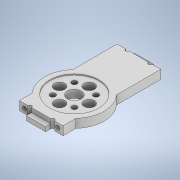
# Autodesk Inventor part: Leg_joint_yaw_frame
Saved by Autodesk Inventor 2020 (Build 240168000, 168)
## iProperties
Created: 2021-10-29
Part Number: Leg_joint_yaw_frame
Material: 一般
Document SubType Name: Modeling
Designer: Masato Kubotera
Density: 1 g/cm^3
Appearance: 既定
Author: Masato Kubotera
Autodesk Inventor part; units mm, degrees
ref_plane "YZ Plane" through (0, 0, 0) normal (1, 0, 0) x (0, 1, 0)
ref_plane "XZ Plane" through (0, 0, 0) normal (0, 1, 0) x (-1, 0, 0)
ref_plane "XY Plane" through (0, 0, 0) normal (0, 0, 1) x (1, 0, 0)
derived "Inner_support_stand.ipt"
sketch "スケッチ1" plane through (0, 0, 0) normal (0, 0, 1) x (1, 0, 0)
  circle A0 centre (0, 0) radius 13.95 construction
  line L0 (0, 13.95) -> (0, -13.95) construction
  circle A1 centre (0, 8.5) radius 1.35 construction
  circle A2 centre (-8.5, 0) radius 1.35 construction
  circle A3 centre (0, -8.5) radius 1.35 construction
  circle A4 centre (8.5, 0) radius 1.35 construction
  circle A5 centre (0, 0) radius 5 construction
  circle A6 centre (0, 0) radius 5.01 construction
  circle A7 centre (-6.1872, 6.1872) radius 2.25 construction
  line L1 (-9.8641, 9.8641) -> (9.8641, -9.8641) construction
  circle A8 centre (-6.1872, 6.1872) radius 1.55
  line L2 (-9.2656, 5.3623) -> (-8.9938, 6.3766) construction
  line L3 (-8.4407, 8.4407) -> (-7.4265, 8.7125) construction
  line L4 (-5.3623, 9.2656) -> (-4.6199, 8.5231) construction
  line L5 (-3.1088, 7.012) -> (-3.3806, 5.9978) construction
  line L6 (-3.9337, 3.9337) -> (-4.9479, 3.6619) construction
  line L7 (-7.012, 3.1088) -> (-7.7545, 3.8513) construction
  circle A9 centre (0, 0) radius 12.49 construction
  arc A10 (-7.4265, 8.7125) -> (-8.7125, 7.4265) centre (-7.6983, 7.6983) ccw construction
  arc A11 (-8.9938, 6.3766) -> (-8.5231, 4.6199) centre (-8.2513, 5.6341) ccw construction
  arc A12 (-7.7545, 3.8513) -> (-5.9978, 3.3806) centre (-6.7403, 4.123) ccw construction
  arc A13 (-4.9479, 3.6619) -> (-3.6619, 4.9479) centre (-4.6761, 4.6761) ccw construction
  arc A14 (-3.3806, 5.9978) -> (-3.8513, 7.7545) centre (-4.123, 6.7403) ccw construction
  arc A15 (-4.6199, 8.5231) -> (-6.3766, 8.9938) centre (-5.6341, 8.2513) ccw construction
  line L8 (-6.3766, 8.9938) -> (-5.3623, 9.2656) construction
  line L9 (-7.4265, 8.7125) -> (-6.3766, 8.9938) construction
  line L10 (-4.6199, 8.5231) -> (-3.8513, 7.7545) construction
  line L11 (-3.8513, 7.7545) -> (-3.1088, 7.012) construction
  line L12 (-3.3806, 5.9978) -> (-3.6619, 4.9479) construction
  line L13 (-3.6619, 4.9479) -> (-3.9337, 3.9337) construction
  line L14 (-4.9479, 3.6619) -> (-5.9978, 3.3806) construction
  line L15 (-5.9978, 3.3806) -> (-7.012, 3.1088) construction
  line L16 (-7.7545, 3.8513) -> (-8.5231, 4.6199) construction
  line L17 (-8.5231, 4.6199) -> (-9.2656, 5.3623) construction
  line L18 (-8.9938, 6.3766) -> (-8.7125, 7.4265) construction
  line L19 (-8.7125, 7.4265) -> (-8.4407, 8.4407) construction
  circle A16 centre (-8.5, 0) radius 2.55 construction
  line L20 (-8.7125, -7.4265) -> (-8.9938, -6.3766) construction
  circle A17 centre (-6.1872, -6.1872) radius 2.25 construction
  circle A18 centre (-6.1872, -6.1872) radius 1.55
  circle A19 centre (0, -8.5) radius 2.55 construction
  arc A20 (-3.8513, -7.7545) -> (-3.3806, -5.9978) centre (-4.123, -6.7403) ccw construction
  line L21 (-3.6619, -4.9479) -> (-3.3806, -5.9978) construction
  arc A21 (-3.6619, -4.9479) -> (-4.9479, -3.6619) centre (-4.6761, -4.6761) ccw construction
  line L22 (-5.9978, -3.3806) -> (-4.9479, -3.6619) construction
  arc A22 (-5.9978, -3.3806) -> (-7.7545, -3.8513) centre (-6.7403, -4.123) ccw construction
  line L23 (-8.5231, -4.6199) -> (-7.7545, -3.8513) construction
  arc A23 (-8.5231, -4.6199) -> (-8.9938, -6.3766) centre (-8.2513, -5.6341) ccw construction
  arc A24 (-8.7125, -7.4265) -> (-7.4265, -8.7125) centre (-7.6983, -7.6983) ccw construction
  line L24 (-6.3766, -8.9938) -> (-7.4265, -8.7125) construction
  arc A25 (-6.3766, -8.9938) -> (-4.6199, -8.5231) centre (-5.6341, -8.2513) ccw construction
  line L25 (-3.8513, -7.7545) -> (-4.6199, -8.5231) construction
  line L26 (7.4265, -8.7125) -> (6.3766, -8.9938) construction
  circle A26 centre (6.1872, -6.1872) radius 2.25 construction
  circle A27 centre (6.1872, -6.1872) radius 1.55
  circle A28 centre (8.5, 0) radius 2.55 construction
  arc A29 (7.7545, -3.8513) -> (5.9978, -3.3806) centre (6.7403, -4.123) ccw construction
  line L27 (4.9479, -3.6619) -> (5.9978, -3.3806) construction
  arc A30 (4.9479, -3.6619) -> (3.6619, -4.9479) centre (4.6761, -4.6761) ccw construction
  line L28 (3.3806, -5.9978) -> (3.6619, -4.9479) construction
  arc A31 (3.3806, -5.9978) -> (3.8513, -7.7545) centre (4.123, -6.7403) ccw construction
  line L29 (4.6199, -8.5231) -> (3.8513, -7.7545) construction
  arc A32 (4.6199, -8.5231) -> (6.3766, -8.9938) centre (5.6341, -8.2513) ccw construction
  arc A33 (7.4265, -8.7125) -> (8.7125, -7.4265) centre (7.6983, -7.6983) ccw construction
  line L30 (8.9938, -6.3766) -> (8.7125, -7.4265) construction
  arc A34 (8.9938, -6.3766) -> (8.5231, -4.6199) centre (8.2513, -5.6341) ccw construction
  line L31 (7.7545, -3.8513) -> (8.5231, -4.6199) construction
  line L32 (8.7125, 7.4265) -> (8.9938, 6.3766) construction
  circle A35 centre (6.1872, 6.1872) radius 2.25 construction
  circle A36 centre (6.1872, 6.1872) radius 1.55
  circle A37 centre (0, 8.5) radius 2.55 construction
  arc A38 (3.8513, 7.7545) -> (3.3806, 5.9978) centre (4.123, 6.7403) ccw construction
  line L33 (3.6619, 4.9479) -> (3.3806, 5.9978) construction
  arc A39 (3.6619, 4.9479) -> (4.9479, 3.6619) centre (4.6761, 4.6761) ccw construction
  line L34 (5.9978, 3.3806) -> (4.9479, 3.6619) construction
  arc A40 (5.9978, 3.3806) -> (7.7545, 3.8513) centre (6.7403, 4.123) ccw construction
  line L35 (8.5231, 4.6199) -> (7.7545, 3.8513) construction
  arc A41 (8.5231, 4.6199) -> (8.9938, 6.3766) centre (8.2513, 5.6341) ccw construction
  arc A42 (8.7125, 7.4265) -> (7.4265, 8.7125) centre (7.6983, 7.6983) ccw construction
  line L36 (6.3766, 8.9938) -> (7.4265, 8.7125) construction
  arc A43 (6.3766, 8.9938) -> (4.6199, 8.5231) centre (5.6341, 8.2513) ccw construction
  line L37 (3.8513, 7.7545) -> (4.6199, 8.5231) construction
  line L38 (-8.8318, 8.8318) -> (-3.5426, 3.5426) construction
  circle A44 centre (0, 0) radius 4
  line L39 (-12.5, -19) -> (-12.5, -11.5954)
  line L40 (-12.5, 37) -> (-7.6, 37)
  line L41 (-12.5, -19) -> (12.5, 37) construction
  line L42 (-12.5, 37) -> (12.5, -19) construction
  arc A45 (-12.5, 11.5954) -> (-12.5, -11.5954) centre (0, 0) ccw
  circle A46 centre (0, 0) radius 14.05
  line L43 (-12.5, 11.5954) -> (-12.5, 37)
  circle A47 centre (0, 8.5) radius 3
  circle A48 centre (-8.5, 0) radius 3
  circle A49 centre (0, -8.5) radius 3
  circle A50 centre (8.5, 0) radius 3
  line L44 (-5.5, -19) -> (-5.5, -22)
  line L45 (-5.5, -22) -> (5.5, -22)
  arc A51 (-5.5, -19) -> (-7.6, -19) centre (-6.55, -19) ccw
  line L46 (-7.6, -19) -> (-12.5, -19)
  line L47 (-5.5, 37) -> (-5.5, 39.9)
  line L48 (-5.5, 39.9) -> (5.5, 39.9)
  arc A52 (-7.6, 37) -> (-5.5, 37) centre (-6.55, 37) ccw
  line L49 (-5.5, -19) -> (5.5, -19)
  line L50 (-5.5, 37) -> (5.5, 37)
  line L51 (0, -22) -> (0, 39.9) construction
  line L52 (12.5, -19) -> (12.5, -11.5954)
  line L53 (12.5, 11.5954) -> (12.5, 37)
  arc A53 (7.6, -19) -> (5.5, -19) centre (6.55, -19) ccw
  arc A54 (5.5, 37) -> (7.6, 37) centre (6.55, 37) ccw
  line L54 (12.5, 37) -> (7.6, 37)
  arc A55 (12.5, -11.5954) -> (12.5, 11.5954) centre (0, 0) ccw
  line L55 (5.5, -19) -> (5.5, -22)
  line L56 (7.6, -19) -> (12.5, -19)
  line L57 (5.5, 37) -> (5.5, 39.9)
  point P0 (-7.012, 3.1088)
  point P1 (-3.9337, 3.9337)
  point P2 (-3.1088, 7.012)
  point P3 (-3.1088, -7.012)
  point P4 (-3.9337, -3.9337)
  point P5 (-7.012, -3.1088)
  point P6 (-9.2656, -5.3623)
  point P7 (-8.4407, -8.4407)
  point P8 (-5.3623, -9.2656)
  point P9 (7.012, -3.1088)
  point P10 (3.9337, -3.9337)
  point P11 (3.1088, -7.012)
  point P12 (5.3623, -9.2656)
  point P13 (8.4407, -8.4407)
  point P14 (9.2656, -5.3623)
  point P15 (3.1088, 7.012)
  point P16 (3.9337, 3.9337)
  point P17 (7.012, 3.1088)
  point P18 (9.2656, 5.3623)
  point P19 (8.4407, 8.4407)
  point P20 (5.3623, 9.2656)
  point P21 (-9.2318, 8.3532)
  point P22 (-9.2318, -8.3532)
  point P23 (-8.3532, -9.2318)
  point P24 (8.3532, -9.2318)
  point P25 (9.2318, -8.3532)
  point P26 (9.2318, 8.3532)
  point P27 (8.3532, 9.2318)
  point P28 (-8.3532, 9.2318)
  point P29 (0, 9)
  dimension "d2" = 25
  dimension "d5" = 3
  dimension "d6" = 0.1
  dimension "d7" = 6
  dimension "d10" = 360
  dimension "d12" = 1.05
  dimension "d13" = 11
  dimension "d14" = 3
  dimension "d15" = 1.05
  dimension "d16" = 2.9
  dimension "d17" = 11
  dimension "d40" = 19
  dimension "d41" = 56
  dimension "d42" = 25
  measures "d2" distance of L40.start L41.end
  measures "d5" radial gap between concentric circles of A45 A46
  measures "d6" radial gap between concentric circles of A46 A0
  measures "d7" diameter of A47
  measures "d12" radius of A51
  measures "d13" distance of L45.end L44.end
  measures "d14" distance of L44.end L44.start
  measures "d15" radius of A52
  measures "d16" distance of L47.start L47.end
  measures "d17" distance of L47.end L48.end
  measures "d40" distance from line of L49 point (0, 0)
  measures "d41" distance between parallel lines of L46 L40
  measures "d42" distance between parallel lines of L52 L39
extrude "押し出し1" add sketch "スケッチ1" along normal blind 5 contours L39 A45 L43 L40 A52 L50 A54 L54 L53 A55 L52 L56 A53 L49 A51 L46
extrude "押し出し2" add sketch "スケッチ1" along normal blind 2.5 contours L49 L55 L45 L44 | L47 L48 L57 L50
extrude "押し出し3" add sketch "スケッチ1" along normal blind 4.5 contours A46
sketch "スケッチ2" plane through (-7.6, -19, 5) normal (0, -1, 0) x (-1, 0, 0)
  line L0 (4.9, 5) -> (0, 5) projected
  line L1 (6.45, 0) -> (-21.65, 0) projected
  line L2 (-7.6, 0) -> (-7.6, 5) construction
  point P0 (1.9, 2.5)
  point P1 (-17.1, 2.5)
  dimension "d24" = 2.5
  dimension "d25" = 19
  constraints: 2 end point, 1 midpoint, 1 symmetric about line, 1 vertical
  measures "d24" distance from line of L0 point (1.9, 2.5)
  measures "d25" distance of point (-17.1, 2.5) point (1.9, 2.5)
hole "穴1" at (-9.5, -19, 2.5) at (9.5, -19, 2.5) direction (0, 1, 0) diameter 2.459 depth 4 tip angle 118 thread size "M3x0.5" class "6H" standard "ISO Metric profile"
sketch "スケッチ3" plane through (7.6, 37, 0) normal (0, 1, 0) x (1, 0, 0)
  circle A0 centre (1.9, -2.5) radius 1.2295 projected
  circle A1 centre (-17.1, -2.5) radius 1.2295 projected
  point P0 (-7.6, 0)
  constraints: 2 coincident
hole "穴2" at (9.5, 37, 2.5) at (-9.5, 37, 2.5) direction (0, -1, 0) diameter 2.459 depth 4 tip angle 118 thread size "M3x0.5" class "6H" standard "ISO Metric profile"
equation "\"d15\" = d12"
